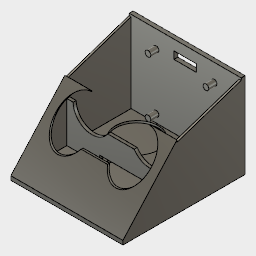
LIDAR Enclosure v2 (Autodesk Fusion 360 design; units mm, degrees)
Autodesk Fusion 360 part; units mm, degrees
sketch "Sketch1" plane through (0, 0, 0) normal (0, 1, 0) x (1, 0, 0)
  line L0 (0, 0) -> (55, 0)
  line L1 (55, 0) -> (55, 60)
  line L2 (55, 60) -> (0, 60)
  line L3 (0, 60) -> (0, 0)
  dimension "d1" = 55
  dimension "d2" = 60
  constraint horizontal L0
  constraint vertical L1
  constraint horizontal L2
  constraint vertical L3
  constraint coincident L0.start L3.end
extrude "Extrude1" add sketch "Sketch1" along normal blind 2
sketch "Sketch2" plane through (0, 2, 0) normal (0, 1, 0) x (-1, 0, 0)
  line L0 (0, -60) -> (0, 0)
  line L1 (0, 0) -> (-55, 0)
  line L2 (-55, 0) -> (-55, -60)
  line L3 (-55, -60) -> (0, -60)
  circle A0 centre (-14.862, -13) radius 10.415
  circle A1 centre (-40.138, -13) radius 10.415
  circle A2 centre (-27.5, -33) radius 10.415
  dimension "d5" = 20.83
  dimension "d6" = 20.83
  dimension "d8" = 14.862
  dimension "d9" = 14.862
  dimension "d10" = 20.83
  dimension "d11" = 27.5
  dimension "d12" = 33
  measures "d5" diameter of A0
  measures "d6" diameter of A1
  measures "d10" diameter of A2
extrude "Extrude2" cut sketch "Sketch2" against normal blind 1 contours A0 | A1 | A2
sketch "Sketch3" plane through (0, 2, 0) normal (0, 1, 0) x (-1, 0, 0)
  circle A0 centre (-27.5, -33) radius 10.415
  circle A1 centre (-40.138, -13) radius 10.415
  circle A2 centre (-14.862, -13) radius 10.415
  line L0 (0, -60) -> (0, 0)
  line L1 (0, 0) -> (-55, 0)
  line L2 (-55, 0) -> (-55, -60)
  line L3 (-55, -60) -> (0, -60)
  line L4 (0, 0) -> (-55, 0)
  line L5 (-55, 0) -> (-55, -2)
  line L6 (-55, -2) -> (0, -2)
  line L7 (0, -2) -> (0, 0)
  dimension "d15" = 2
  constraint horizontal L4
  constraint vertical L5
  constraint horizontal L6
  constraint vertical L7
  constraint coincident L2 L0.end
  constraint coincident L0.end L1.start
extrude "Extrude3" add sketch "Sketch3" along normal blind 40 contours L0 L1 L2 L4 L5 L6 L7
sketch "Sketch4" plane through (0, 0, -2) normal (0, 0, -1) x (-1, 0, 0)
  line L0 (-55, 2) -> (0, 2)
  line L1 (0, 2) -> (0, 42)
  line L2 (0, 42) -> (-55, 42)
  line L3 (-55, 42) -> (-55, 2)
  circle A0 centre (-41.724, 6) radius 1.4
  circle A1 centre (-13.276, 6) radius 1.4
  circle A2 centre (-41.7224, 33.432) radius 1.4
  circle A3 centre (-13.276, 33.432) radius 1.4
  dimension "d18" = 2.8
  dimension "d19" = 2.8
  dimension "d20" = 2.8
  dimension "d21" = 2.8
  dimension "d22" = 27.432
  dimension "d23" = 28.448
  dimension "d24" = 27.432
  dimension "d26" = 27.432
  dimension "d27" = 28.448
  dimension "d28" = 4
  dimension "d29" = 13.276
  measures "d18" diameter of A0
  measures "d19" diameter of A1
  measures "d20" diameter of A2
  measures "d21" diameter of A3
  measures "d22" distance of origin
  measures "d23" distance of origin
  measures "d27" distance of origin
  measures "d29" distance of L3 origin
extrude "Extrude4" add sketch "Sketch4" along normal blind 4 contours A0 | A1 | A2 | A3
sketch "Sketch5" plane through (0, 2, 0) normal (0, 1, 0) x (-1, 0, 0)
  line L0 (0, -2) -> (-55, -2)
  line L1 (-55, -2) -> (-55, -60)
  line L2 (-55, -60) -> (0, -60)
  line L3 (0, -60) -> (0, -2)
  circle A0 centre (-27.5, -33) radius 10.415
  circle A1 centre (-40.138, -13) radius 10.415
  circle A2 centre (-14.862, -13) radius 10.415
  line L4 (0, -32) -> (-55, -32)
  line L5 (-55, -32) -> (-55, -33.5)
  line L6 (-55, -33.5) -> (0, -33.5)
  line L7 (0, -33.5) -> (0, -32)
  dimension "d32" = 1.5
  dimension "d33" = 30
  constraint horizontal L4
  constraint vertical L5
  constraint horizontal L6
  constraint vertical L7
  constraint coincident L1 origin
  constraint coincident L3 origin
  measures "d33" distance of L0 L4
extrude "Extrude5" add sketch "Sketch5" along normal blind 20 contours L3 A0 L4 L6 L7 | L1 A0 L4 L5 L6 | A0 L4 L6
extrude "Extrude6" cut sketch "Sketch2" along normal blind 4 contours A2
sketch "Sketch6" plane through (0, 0, -33.5) normal (0, 0, -1) x (-1, 0, 0)
  line L0 (-37.903, 2) -> (-37.903, 6)
  line L1 (-37.903, 6) -> (-17.097, 6)
  line L2 (-17.097, 6) -> (-17.097, 2)
  line L3 (-17.097, 2) -> (0, 2)
  line L4 (0, 2) -> (0, 22)
  line L5 (0, 22) -> (-55, 22)
  line L6 (-55, 22) -> (-55, 2)
  line L7 (-55, 2) -> (-37.903, 2)
  line L8 (-55, 42) -> (-55, 2)
  line L9 (0, 2) -> (0, 42)
  line L10 (-32.524, 22) -> (-22.476, 22)
  line L11 (-20.9987, 17) -> (-34.0013, 17)
  arc A0 (-32.524, 22) -> (-34.0013, 17) centre (-41.724, 22) ccw
  arc A1 (-20.9987, 17) -> (-22.476, 22) centre (-13.276, 22) ccw
  dimension "d38" = 18.4
  dimension "d40" = 18.4
  dimension "d41" = 13.276
  dimension "d42" = 13.276
  constraint midpoint L5 origin
  constraint coincident L5 origin
  constraint horizontal L10
  constraint horizontal L11
  measures "d38" diameter of A0
  measures "d40" diameter of A1
  measures "d41" distance of origin L8
  measures "d42" distance of origin L9
extrude "Extrude7" cut sketch "Sketch6" against normal blind 2 contours L5 L10 L11 A0 A1
sketch "Sketch7" plane through (0, 0, 0) normal (-1, 0, 0) x (0, 0, 1)
  line L0 (-60, 0) -> (0, 0)
  line L1 (0, 0) -> (0, 42)
  line L2 (0, 42) -> (-2, 42)
  line L3 (-2, 42) -> (-2, 2)
  line L4 (-2, 2) -> (-32, 2)
  line L5 (-32, 2) -> (-32, 22)
  line L6 (-32, 22) -> (-33.5, 22)
  line L7 (-33.5, 22) -> (-33.5, 2)
  line L8 (-33.5, 2) -> (-60, 2)
  line L9 (-60, 2) -> (-60, 0)
  line L10 (-33.5, 31.4252) -> (-60, 2)
  line L11 (-33.5, 31.2) -> (-33.5, 12.8)
  line L12 (-33.5, 2) -> (-33.5, 42)
  line L13 (-33.5, 30.4252) -> (-59, 2)
  dimension "d46" = 1
  dimension "d47" = 1
  constraint coincident L0.end L1.start
  constraint coincident L11 L0.end
  constraint coincident L8 L0.end
  measures "d46" distance of L0.end
extrude "Extrude8" add sketch "Sketch7" against normal blind 55 contours L8 L10 L11 L12 L13
sketch "Sketch8" plane through (0, 0, 0) normal (-1, 0, 0) x (0, 0, 1)
  line L0 (-60, 0) -> (0, 0)
  line L1 (0, 0) -> (0, 42)
  line L2 (0, 42) -> (-2, 42)
  line L3 (-2, 42) -> (-2, 2)
  line L4 (-2, 2) -> (-32, 2)
  line L5 (-32, 2) -> (-32, 22)
  line L6 (-32, 22) -> (-33.5, 22)
  line L7 (-33.5, 22) -> (-33.5, 2)
  line L8 (-33.5, 2) -> (-59, 2)
  line L9 (-59, 2) -> (-33.5, 30.4252)
  line L10 (-33.5, 30.4252) -> (-33.5, 31.4252)
  line L11 (-33.5, 31.4252) -> (-60, 2)
  line L12 (-60, 2) -> (-60, 0)
  line L13 (-60, 0) -> (-60, 2)
  line L14 (-60, 0) -> (0, 0)
  line L15 (-2, 41) -> (-33.5, 30.4252)
  dimension "d52" = 1
  constraint coincident L0.end L1.start
  constraint coincident L3 L0.end
  measures "d52" distance of L0.end
extrude "Extrude10" add sketch "Sketch8" against normal blind 1 contours L3 L4 L5 L6 L7 L8 L9 L15
sketch "Sketch9" plane through (55, 0, 0) normal (1, 0, 0) x (0, 0, -1)
  line L0 (0, 0) -> (60, 0)
  line L1 (60, 0) -> (60, 2)
  line L2 (60, 2) -> (33.5, 31.4252)
  line L3 (33.5, 31.4252) -> (33.5, 30.4252)
  line L4 (33.5, 30.4252) -> (59, 2)
  line L5 (59, 2) -> (33.5, 2)
  line L6 (33.5, 2) -> (32, 2)
  line L7 (32, 2) -> (2, 2)
  line L8 (2, 2) -> (2, 42)
  line L9 (2, 42) -> (0, 42)
  line L10 (0, 42) -> (0, 0)
  line L11 (2, 41) -> (33.5, 30.4252)
  line L12 (2, 41) -> (2, 2)
  line L13 (59, 2) -> (2, 2)
  line L14 (59, 2) -> (33.5, 30.4252)
  dimension "d55" = 1
  constraint coincident L8
  constraint coincident L0.start L10.end
  measures "d55" distance of L9
extrude "Extrude11" add sketch "Sketch9" against normal blind 1 contours L4 L5 L6 L7 L8 L11 L12 L13 L14
extrude "Extrude12" cut sketch "Sketch6" along normal blind 20 contours L5 A0 | L5 L10 L11 A0 A1 | L5 A1
sketch "Sketch10" plane through (0, 30.732, -34.1243) normal (0, 0.669206, -0.743077) x (-1, 0, 0)
  line L0 (-32.524, -11.7511) -> (-22.476, -11.7511)
  ellipse E0 centre (-13.276, -11.7511) end of major axis (-13.276, -24.132) minor radius 9.2 (-20.9987, -18.4799) -> (-22.476, -11.7511) ccw
  line L1 (-20.9987, -18.4799) -> (-34.0013, -18.4799)
  ellipse E1 centre (-41.724, -11.7511) end of major axis (-41.724, 0.6299) minor radius 9.2 (-32.524, -11.7511) -> (-34.0013, -18.4799) ccw
  line L2 (0, -38.6662) -> (0, 0.933)
  line L3 (0, 0.933) -> (-55, 0.933)
  line L4 (-55, 0.933) -> (-55, -38.6662)
  line L5 (-55, -38.6662) -> (0, -38.6662)
  line L6 (-41.724, 0.6299) -> (-41.724, 0.933)
  line L7 (-13.276, 0.933) -> (-13.276, 0.6299)
  dimension "d61" = 13.276
  dimension "d62" = 13.276
  dimension "d63" = 13.276
  dimension "d64" = 13.276
  constraint coincident L3
  constraint coincident E1 origin
  constraint coincident E0 origin
  measures "d61" distance of L4
  measures "d62" distance of L4 origin
  measures "d63" distance of L2
  measures "d64" distance of L2 origin
extrude "Extrude13" cut sketch "Sketch10" against normal blind 2 contours L0 E0 E1 L3 L6 L7
sketch "Sketch11" plane through (0, 0, -2) normal (0, 0, -1) x (-1, 0, 0)
  circle A0 centre (-13.276, 33.432) radius 1.4
  circle A1 centre (-13.276, 6) radius 1.4
  circle A2 centre (-41.7224, 33.432) radius 1.4
  circle A3 centre (-41.724, 6) radius 1.4
  line L0 (-55, 41) -> (-54, 41)
  line L1 (-54, 41) -> (-54, 2)
  line L2 (-54, 2) -> (-1, 2)
  line L3 (-1, 2) -> (-1, 41)
  line L4 (-1, 41) -> (0, 41)
  line L5 (0, 41) -> (0, 42)
  line L6 (0, 42) -> (-55, 42)
  line L7 (-55, 42) -> (-55, 41)
  line L8 (-33, 37) -> (-22, 37)
  line L9 (-22, 37) -> (-22, 33.3725)
  line L10 (-22, 33.3725) -> (-33, 33.3725)
  line L11 (-33, 33.3725) -> (-33, 37)
  dimension "d67" = 21
  dimension "d68" = 21
  constraint horizontal L8
  constraint vertical L9
  constraint horizontal L10
  constraint vertical L11
  measures "d67" distance of L1 L11
  measures "d68" distance of L3 L9
extrude "Extrude14" cut sketch "Sketch11" against normal blind 14 contours L8 L9 L10 L11
equation "d8 = 4.447 mm + ( 20.83 / 2 ) * 1 mm"
equation "d9 = 4.447 mm + ( 20.83 / 2 ) * 1 mm"
equation "d11 = ( 55 / 2 ) * 1 mm"
equation "d38 = ( 18.4 ) * 1 mm"
